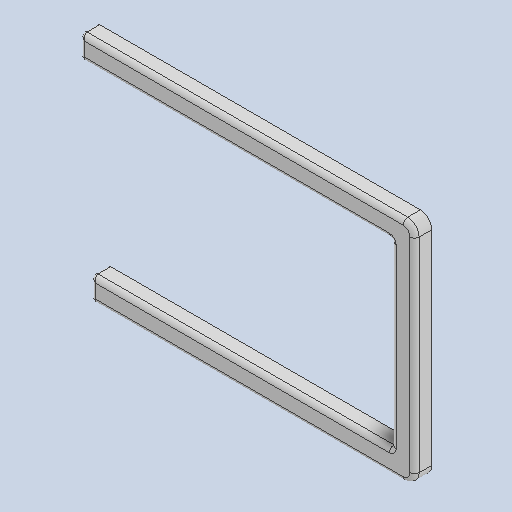
# Autodesk Inventor part: Top_Right
Saved by Autodesk Inventor 2023 (Build 270158000, 158)
## iProperties
Created: 2022-11-13
Part Number: Top_Right
Material: Generic
Document SubType Name: Modeling
Designer: reide
Density: 1 g/cm^3
Appearance: Default
Author: reide
Autodesk Inventor part; units mm, degrees
ref_plane "YZ Plane" through (0, 0, 0) normal (1, 0, 0) x (0, 1, 0)
ref_plane "XZ Plane" through (0, 0, 0) normal (0, 1, 0) x (-1, 0, 0)
ref_plane "XY Plane" through (0, 0, 0) normal (0, 0, 1) x (1, 0, 0)
sketch "Sketch1" plane through (0, 0, 0) normal (0, 0, 1) x (1, 0, 0)
  line L0 (-55.675, 43.6202) -> (-45.6, 43.6202)
  arc A0 (-46.5875, 44.4623) -> (-45.6, 43.6202) centre (-45.6, 44.6202) ccw
  ellipse E0 centre (-45.6, 44.2959) end of major axis (-45.6, 43.2418) minor radius 1 (-45.6, 45.35) -> (-46.5875, 44.4623) ccw
  line L1 (-45.6, 45.35) -> (-32.6, 45.35)
  ellipse E1 centre (-32.6, 44.2959) end of major axis (-32.6, 43.2418) minor radius 1 (-31.6, 44.2959) -> (-32.6, 45.35) ccw
  line L2 (-31.6, 42.35) -> (-31.6, 44.2959)
  arc A1 (-32.6, 41.35) -> (-31.6, 42.35) centre (-32.6, 42.35) ccw
  line L3 (-32.6, 41.35) -> (-37.675, 41.35)
  arc A2 (-38.675, 42.35) -> (-37.675, 41.35) centre (-37.675, 42.35) ccw
  line L4 (-38.675, 42.35) -> (-38.675, 40.35)
  arc A3 (-38.675, 40.35) -> (-37.675, 39.35) centre (-37.675, 40.35) ccw
  line L5 (-37.675, 39.35) -> (-31.6, 39.35)
  line L6 (-31.6, 39.35) -> (-31.6, 41.65)
  arc A4 (-30.6, 42.65) -> (-31.6, 41.65) centre (-30.6, 41.65) ccw
  line L7 (-30.6, 42.65) -> (-12, 42.65)
  arc A5 (-11, 41.65) -> (-12, 42.65) centre (-12, 41.65) ccw
  line L8 (-11, 41.65) -> (-11, 39.35)
  line L9 (-11, 39.35) -> (25.55, 39.35)
  line L10 (25.55, 39.35) -> (25.55, 41.65)
  arc A6 (26.55, 42.65) -> (25.55, 41.65) centre (26.55, 41.65) ccw
  line L11 (26.55, 42.65) -> (45.15, 42.65)
  arc A7 (46.15, 41.65) -> (45.15, 42.65) centre (45.15, 41.65) ccw
  line L12 (46.15, 41.65) -> (46.15, 39.35)
  line L13 (46.15, 39.35) -> (61.675, 39.35)
  arc A8 (62.675, 38.35) -> (61.675, 39.35) centre (61.675, 38.35) ccw
  line L14 (62.675, 38.35) -> (62.675, 15.986)
  arc A9 (62.675, 15.986) -> (63.675, 14.986) centre (63.675, 15.986) ccw
  line L15 (63.675, 14.986) -> (66.925, 14.986)
  line L16 (66.925, 14.986) -> (66.925, 14.8578)
  spline S0 degree 3 poles (66.925, 14.8578) (66.925, 14.7146) (66.9302, 14.5854) (66.9421, 14.2499) (66.9452, 14.1381) (66.9452, 13.986) knots 0 0 0 0 0.477344 0.477344 1 1 1 1
  line L17 (66.9452, 13.986) -> (66.9452, 2.986)
  spline S1 degree 3 poles (66.9452, 2.986) (66.9452, 2.8339) (66.9421, 2.7221) (66.9302, 2.3866) (66.925, 2.2574) (66.925, 2.1142) knots 0 0 0 0 0.522656 0.522656 1 1 1 1
  line L18 (66.925, 2.1142) -> (66.925, 1.986)
  line L19 (66.925, 1.986) -> (63.675, 1.986)
  arc A10 (63.675, 1.986) -> (62.675, 0.986) centre (63.675, 0.986) ccw
  line L20 (62.675, 0.986) -> (62.675, -2.225)
  line L21 (62.675, -2.225) -> (64.975, -2.225)
  arc A11 (65.975, -3.225) -> (64.975, -2.225) centre (64.975, -3.225) ccw
  line L22 (65.975, -3.225) -> (65.975, -21.825)
  arc A12 (64.975, -22.825) -> (65.975, -21.825) centre (64.975, -21.825) ccw
  line L23 (64.975, -22.825) -> (62.675, -22.825)
  line L24 (62.675, -22.825) -> (62.675, -38.35)
  arc A13 (61.675, -39.35) -> (62.675, -38.35) centre (61.675, -38.35) ccw
  line L25 (61.675, -39.35) -> (46.15, -39.35)
  line L26 (46.15, -39.35) -> (46.15, -41.65)
  arc A14 (45.15, -42.65) -> (46.15, -41.65) centre (45.15, -41.65) ccw
  line L27 (45.15, -42.65) -> (26.55, -42.65)
  arc A15 (25.55, -41.65) -> (26.55, -42.65) centre (26.55, -41.65) ccw
  line L28 (25.55, -41.65) -> (25.55, -39.35)
  line L29 (25.55, -39.35) -> (-31.2875, -39.35)
  line L30 (-31.2875, -39.35) -> (-31.2875, -41.65)
  arc A16 (-32.2875, -42.65) -> (-31.2875, -41.65) centre (-32.2875, -41.65) ccw
  line L31 (-32.2875, -42.65) -> (-50.8875, -42.65)
  arc A17 (-51.8875, -41.65) -> (-50.8875, -42.65) centre (-50.8875, -41.65) ccw
  line L32 (-51.8875, -41.65) -> (-51.8875, -39.35)
  line L33 (-51.8875, -39.35) -> (-66.9125, -39.35)
  arc A18 (-66.9125, -39.35) -> (-67.9125, -40.35) centre (-66.9125, -40.35) ccw
  line L34 (-67.9125, -40.35) -> (-67.9125, -48.35)
  arc A19 (-67.9125, -48.35) -> (-66.9125, -49.35) centre (-66.9125, -48.35) ccw
  line L35 (-66.9125, -49.35) -> (67.675, -49.35)
  arc A20 (67.675, -49.35) -> (72.675, -44.35) centre (67.675, -44.35) ccw
  line L36 (72.675, -44.35) -> (72.675, 44.35)
  arc A21 (72.675, 44.35) -> (67.675, 49.35) centre (67.675, 44.35) ccw
  line L37 (67.675, 49.35) -> (-71.675, 49.35)
  arc A22 (-71.675, 49.35) -> (-72.675, 48.35) centre (-71.675, 48.35) ccw
  line L38 (-72.675, 48.35) -> (-72.675, 40.35)
  arc A23 (-72.675, 40.35) -> (-71.675, 39.35) centre (-71.675, 40.35) ccw
  line L39 (-71.675, 39.35) -> (-57.675, 39.35)
  arc A24 (-57.675, 39.35) -> (-56.675, 40.35) centre (-57.675, 40.35) ccw
  line L40 (-56.675, 40.35) -> (-56.675, 43.6)
  line L41 (-56.675, 43.6) -> (-56.5468, 43.6)
  spline S2 degree 3 poles (-56.5468, 43.6) (-56.4036, 43.6) (-56.2744, 43.6052) (-55.9389, 43.6171) (-55.8271, 43.6202) (-55.675, 43.6202) knots 0 0 0 0 0.477344 0.477344 1 1 1 1
  line L42 (47.15, -41.35) -> (60.15, -41.35)
  arc A25 (61.15, -42.35) -> (60.15, -41.35) centre (60.15, -42.35) ccw
  line L43 (61.15, -44.2959) -> (61.15, -42.35)
  ellipse E2 centre (60.15, -44.2959) end of major axis (60.15, -43.2418) minor radius 1 (60.15, -45.35) -> (61.15, -44.2959) ccw
  line L44 (60.15, -45.35) -> (47.15, -45.35)
  ellipse E3 centre (47.15, -44.2959) end of major axis (47.15, -43.2418) minor radius 1 (46.15, -44.2959) -> (47.15, -45.35) ccw
  line L45 (46.15, -42.35) -> (46.15, -44.2959)
  arc A26 (47.15, -41.35) -> (46.15, -42.35) centre (47.15, -42.35) ccw
  line L46 (-30.2875, -41.35) -> (-17.2875, -41.35)
  arc A27 (-16.2875, -42.35) -> (-17.2875, -41.35) centre (-17.2875, -42.35) ccw
  line L47 (-16.2875, -44.2959) -> (-16.2875, -42.35)
  ellipse E4 centre (-17.2875, -44.2959) end of major axis (-17.2875, -43.2418) minor radius 1 (-17.2875, -45.35) -> (-16.2875, -44.2959) ccw
  line L48 (-17.2875, -45.35) -> (-30.2875, -45.35)
  ellipse E5 centre (-30.2875, -44.2959) end of major axis (-30.2875, -43.2418) minor radius 1 (-31.2875, -44.2959) -> (-30.2875, -45.35) ccw
  line L49 (-31.2875, -42.35) -> (-31.2875, -44.2959)
  arc A28 (-30.2875, -41.35) -> (-31.2875, -42.35) centre (-30.2875, -42.35) ccw
  circle A29 centre (-62.9125, -44.35) radius 2.125
  circle A30 centre (67.675, -44.35) radius 2.125
  circle A31 centre (-67.675, 44.35) radius 2.125
  circle A32 centre (67.675, 44.35) radius 2.125
  arc A33 (46.15, 42.35) -> (47.15, 41.35) centre (47.15, 42.35) ccw
  line L50 (46.15, 44.2959) -> (46.15, 42.35)
  ellipse E6 centre (47.15, 44.2959) end of major axis (47.15, 43.2418) minor radius 1 (47.15, 45.35) -> (46.15, 44.2959) ccw
  line L51 (47.15, 45.35) -> (60.15, 45.35)
  ellipse E7 centre (60.15, 44.2959) end of major axis (60.15, 43.2418) minor radius 1 (61.15, 44.2959) -> (60.15, 45.35) ccw
  line L52 (61.15, 42.35) -> (61.15, 44.2959)
  arc A34 (60.15, 41.35) -> (61.15, 42.35) centre (60.15, 42.35) ccw
  line L53 (60.15, 41.35) -> (47.15, 41.35)
  line L54 (-57.675, 39.35) -> (46.15, 39.35)
  line L55 (62.675, 15.986) -> (62.675, -22.825)
  line L56 (46.15, -39.35) -> (-51.8875, -39.35)
  point P0 (0, 0)
  constraints: 6 end point, 2 perpendicular, 1 horizontal, 8 other
extrude "Extrusion1" add sketch "Sketch1" along normal blind 7.5 contours S2 L41 L40 A24 L39 A23 L38 A22 L37 A21 L36 A20 L35 A19 L34 A18 L33 L32 A17 L31 A16 L30 L29 L28 A15 L27 A14 L26 L25 A13 L24 L23 A12 L22 A11 L21 L20 A10 L19 L18 S1 L17 S0 L16 L15 A9 L14 A8 L13 L12 A7 L11 A6 L10 L9 L8 A5 L7 A4 L6 L5 A3 L4 A2 L3 A1 L2 E1 L1 E0 A0 L0 | L0 A0 E0 L1 E1 L2 A1 L3 A2 L4 A3 L54 A24 L40 L41 S2 | L6 A4 L7 A5 L8 L54 | L10 A6 L11 A7 L12 L54 | A9 L15 L16 S0 L17 S1 L18 L19 A10 L55 | L21 A11 L22 A12 L23 L55 | L56 L30 A16 L31 A17 L32 | L26 A14 L27 A15 L28 L56 | L42 A25 L43 E2 L44 E3 L45 A26 | L46 A27 L47 E4 L48 E5 L49 A28 | A29 | A30 | A31 | A32 | L50 E6 L51 E7 L52 A34 L53 A33
fillet "Fillet1" radius 2 30 edges at (62.3821, 39.0571, 7.5) (62.675, -30.5875, 7.5) (62.675, -12.525, 7.5) (62.675, -0.6195, 7.5) (62.675, 8.486, 7.5) (62.675, 27.168, 7.5) (62.3821, -39.0571, 7.5) (-59.4, -39.35, 7.5) (-41.5875, -39.35, 7.5) (-2.8687, -39.35, 7.5) (35.85, -39.35, 7.5) (53.9125, -39.35, 7.5) (-67.6196, -39.6429, 7.5) (-67.9125, -44.35, 7.5) (-67.6196, -49.0571, 7.5) (0.3813, -49.35, 7.5) (71.2105, -47.8855, 7.5) (72.675, 0, 7.5) (71.2105, 47.8855, 7.5) (-2, 49.35, 7.5) (-72.3821, 49.0571, 7.5) (-72.675, 44.35, 7.5) (-72.3821, 39.6429, 7.5) (7.275, 39.35, 7.5) (-21.3, 39.35, 7.5) (-34.6375, 39.35, 7.5) (-47.675, 39.35, 7.5) (-64.675, 39.35, 7.5) (53.9125, 39.35, 7.5) (35.85, 39.35, 7.5)
sketch "Sketch3" plane through (-72.675, 40.35, 0) normal (-1, 0, 0) x (0, 0, 1)
  line L0 (0, -40.35) -> (17.2642, -40.35)
  line L1 (0.1, -1) -> (5.6, -1) projected
  line L2 (0.1, 9) -> (5.6, 9) projected
  line L3 (0, -84.7) -> (0, 4) projected
  line L4 (0, -1) -> (5.5, -1) projected
  line L5 (0, -1) -> (0, 1)
  line L6 (0, 1) -> (3, 1)
  line L7 (3, 1) -> (3, 6.3)
  line L8 (0, 1) -> (0, 5.3)
  line L9 (0, 5.3) -> (3, 6.3)
  line L10 (0.1, -79.7) -> (5.6, -79.7)
  line L11 (0, 4) -> (0, -84.7)
  line L12 (0, -79.7) -> (5.5, -79.7)
  line L13 (0, -79.7) -> (0, -81.7)
  line L14 (0, -81.7) -> (3, -81.7)
  line L15 (3, -81.7) -> (3, -87)
  line L16 (0, -81.7) -> (0, -86)
  line L17 (0, -82.575) -> (0, -86.825)
  line L18 (0, -86) -> (3, -87)
  point P0 (0, 1.875)
  point P1 (0, 1)
  dimension "d11" = 2
  dimension "d12" = 3
  dimension "d13" = 5.3
  dimension "d14" = 4.3
  constraints: 30 end point, 11 symmetric about line, 1 horizontal, 1 perpendicular, 1 point on line, 1 vertical
  measures "d11" distance of L4.start L5.end
  measures "d12" distance of L5.end L6.end
  measures "d13" distance of L6.end L7.end
  measures "d14" distance of L5.end L8.end
extrude "Extrusion3" cut sketch "Sketch3" against normal up to surface (145.35 mm away)
sketch "Sketch4" plane through (0, 0, 0) normal (0, 0, -1) x (-1, 0, 0)
  line L0 (55.675, 43.605) -> (45.6, 43.605)
  arc A0 (45.6, 43.605) -> (46.5886, 44.4545) centre (45.6, 44.605) ccw
  ellipse E0 centre (45.6, 44.2959) end of major axis (45.6, 43.2418) minor radius 1 (46.5886, 44.4545) -> (45.6, 45.35) ccw
  line L1 (45.6, 45.35) -> (32.6, 45.35)
  ellipse E1 centre (32.6, 44.2959) end of major axis (32.6, 43.2418) minor radius 1 (32.6, 45.35) -> (31.6, 44.2959) ccw
  line L2 (31.6, 42.35) -> (31.6, 44.2959)
  arc A1 (31.6, 42.35) -> (32.6, 41.35) centre (32.6, 42.35) ccw
  line L3 (32.6, 41.35) -> (37.675, 41.35)
  arc A2 (37.675, 41.35) -> (38.675, 42.35) centre (37.675, 42.35) ccw
  line L4 (38.675, 42.35) -> (38.675, 40.35)
  arc A3 (37.675, 39.35) -> (38.675, 40.35) centre (37.675, 40.35) ccw
  line L5 (37.675, 39.35) -> (31.6, 39.35)
  line L6 (31.6, 39.35) -> (31.6, 41.65)
  arc A4 (31.6, 41.65) -> (30.6, 42.65) centre (30.6, 41.65) ccw
  line L7 (30.6, 42.65) -> (12, 42.65)
  arc A5 (12, 42.65) -> (11, 41.65) centre (12, 41.65) ccw
  line L8 (11, 41.65) -> (11, 39.35)
  line L9 (11, 39.35) -> (-25.55, 39.35)
  line L10 (-25.55, 39.35) -> (-25.55, 41.65)
  arc A6 (-25.55, 41.65) -> (-26.55, 42.65) centre (-26.55, 41.65) ccw
  line L11 (-26.55, 42.65) -> (-45.15, 42.65)
  arc A7 (-45.15, 42.65) -> (-46.15, 41.65) centre (-45.15, 41.65) ccw
  line L12 (-46.15, 41.65) -> (-46.15, 39.35)
  line L13 (-46.15, 39.35) -> (-61.675, 39.35)
  arc A8 (-61.675, 39.35) -> (-62.675, 38.35) centre (-61.675, 38.35) ccw
  line L14 (-62.675, 38.35) -> (-62.675, 15.986)
  arc A9 (-63.675, 14.986) -> (-62.675, 15.986) centre (-63.675, 15.986) ccw
  line L15 (-63.675, 14.986) -> (-66.925, 14.986)
  line L16 (-66.925, 14.986) -> (-66.925, 14.6105)
  spline S0 degree 3 poles (-66.925, 14.6105) (-66.925, 14.5088) (-66.9263, 14.4189) (-66.9292, 14.1781) (-66.93, 14.0946) (-66.93, 13.986) knots 0 0 0 0 0.491042 0.491042 1 1 1 1
  line L17 (-66.93, 13.986) -> (-66.93, 2.986)
  spline S1 degree 3 poles (-66.93, 2.986) (-66.93, 2.8774) (-66.9292, 2.7939) (-66.9263, 2.5531) (-66.925, 2.4632) (-66.925, 2.3615) knots 0 0 0 0 0.508958 0.508958 1 1 1 1
  line L18 (-66.925, 2.3615) -> (-66.925, 1.986)
  line L19 (-66.925, 1.986) -> (-63.675, 1.986)
  arc A10 (-62.675, 0.986) -> (-63.675, 1.986) centre (-63.675, 0.986) ccw
  line L20 (-62.675, 0.986) -> (-62.675, -2.225)
  line L21 (-62.675, -2.225) -> (-64.975, -2.225)
  arc A11 (-64.975, -2.225) -> (-65.975, -3.225) centre (-64.975, -3.225) ccw
  line L22 (-65.975, -3.225) -> (-65.975, -21.825)
  arc A12 (-65.975, -21.825) -> (-64.975, -22.825) centre (-64.975, -21.825) ccw
  line L23 (-64.975, -22.825) -> (-62.675, -22.825)
  line L24 (-62.675, -22.825) -> (-62.675, -38.35)
  arc A13 (-62.675, -38.35) -> (-61.675, -39.35) centre (-61.675, -38.35) ccw
  line L25 (-61.675, -39.35) -> (-46.15, -39.35)
  line L26 (-46.15, -39.35) -> (-46.15, -41.65)
  arc A14 (-46.15, -41.65) -> (-45.15, -42.65) centre (-45.15, -41.65) ccw
  line L27 (-45.15, -42.65) -> (-26.55, -42.65)
  arc A15 (-26.55, -42.65) -> (-25.55, -41.65) centre (-26.55, -41.65) ccw
  line L28 (-25.55, -41.65) -> (-25.55, -39.35)
  line L29 (-25.55, -39.35) -> (31.2875, -39.35)
  line L30 (31.2875, -39.35) -> (31.2875, -41.65)
  arc A16 (31.2875, -41.65) -> (32.2875, -42.65) centre (32.2875, -41.65) ccw
  line L31 (32.2875, -42.65) -> (50.8875, -42.65)
  arc A17 (50.8875, -42.65) -> (51.8875, -41.65) centre (50.8875, -41.65) ccw
  line L32 (51.8875, -41.65) -> (51.8875, -39.35)
  line L33 (51.8875, -39.35) -> (66.9125, -39.35)
  arc A18 (67.9125, -40.35) -> (66.9125, -39.35) centre (66.9125, -40.35) ccw
  line L34 (67.9125, -40.35) -> (67.9125, -48.35)
  arc A19 (66.9125, -49.35) -> (67.9125, -48.35) centre (66.9125, -48.35) ccw
  line L35 (66.9125, -49.35) -> (-67.675, -49.35)
  arc A20 (-72.675, -44.35) -> (-67.675, -49.35) centre (-67.675, -44.35) ccw
  line L36 (-72.675, -44.35) -> (-72.675, 44.35)
  arc A21 (-67.675, 49.35) -> (-72.675, 44.35) centre (-67.675, 44.35) ccw
  line L37 (-67.675, 49.35) -> (71.675, 49.35)
  arc A22 (72.675, 48.35) -> (71.675, 49.35) centre (71.675, 48.35) ccw
  line L38 (72.675, 48.35) -> (72.675, 40.35)
  arc A23 (71.675, 39.35) -> (72.675, 40.35) centre (71.675, 40.35) ccw
  line L39 (71.675, 39.35) -> (57.675, 39.35)
  arc A24 (56.675, 40.35) -> (57.675, 39.35) centre (57.675, 40.35) ccw
  line L40 (56.675, 40.35) -> (56.675, 43.6)
  line L41 (56.675, 43.6) -> (56.2995, 43.6)
  spline S2 degree 3 poles (56.2995, 43.6) (56.1978, 43.6) (56.1079, 43.6013) (55.8671, 43.6042) (55.7836, 43.605) (55.675, 43.605) knots 0 0 0 0 0.491042 0.491042 1 1 1 1
  line L42 (-47.15, -41.3502) -> (-60.15, -41.3502)
  arc A25 (-60.15, -41.3502) -> (-61.15, -42.3502) centre (-60.15, -42.3502) ccw
  line L43 (-61.15, -44.2961) -> (-61.15, -42.3502)
  ellipse E2 centre (-60.15, -44.2961) end of major axis (-60.15, -43.242) minor radius 1 (-61.15, -44.2961) -> (-60.15, -45.3502) ccw
  line L44 (-60.15, -45.3502) -> (-47.15, -45.3502)
  ellipse E3 centre (-47.15, -44.2961) end of major axis (-47.15, -43.242) minor radius 1 (-47.15, -45.3502) -> (-46.15, -44.2961) ccw
  line L45 (-46.15, -42.3502) -> (-46.15, -44.2961)
  arc A26 (-46.15, -42.3502) -> (-47.15, -41.3502) centre (-47.15, -42.3502) ccw
  line L46 (30.2875, -41.3502) -> (17.2875, -41.3502)
  arc A27 (17.2875, -41.3502) -> (16.2875, -42.3502) centre (17.2875, -42.3502) ccw
  line L47 (16.2875, -44.2961) -> (16.2875, -42.3502)
  ellipse E4 centre (17.2875, -44.2961) end of major axis (17.2875, -43.242) minor radius 1 (16.2875, -44.2961) -> (17.2875, -45.3502) ccw
  line L48 (17.2875, -45.3502) -> (30.2875, -45.3502)
  ellipse E5 centre (30.2875, -44.2961) end of major axis (30.2875, -43.242) minor radius 1 (30.2875, -45.3502) -> (31.2875, -44.2961) ccw
  line L49 (31.2875, -42.3502) -> (31.2875, -44.2961)
  arc A28 (31.2875, -42.3502) -> (30.2875, -41.3502) centre (30.2875, -42.3502) ccw
  circle A29 centre (62.9125, -44.35) radius 2.125
  circle A30 centre (-67.675, -44.35) radius 2.125
  circle A31 centre (67.675, 44.35) radius 2.125
  circle A32 centre (-67.675, 44.35) radius 2.125
  arc A33 (-47.15, 41.35) -> (-46.15, 42.35) centre (-47.15, 42.35) ccw
  line L50 (-46.15, 44.2959) -> (-46.15, 42.35)
  ellipse E6 centre (-47.15, 44.2959) end of major axis (-47.15, 43.2418) minor radius 1 (-46.15, 44.2959) -> (-47.15, 45.35) ccw
  line L51 (-47.15, 45.35) -> (-60.15, 45.35)
  ellipse E7 centre (-60.15, 44.2959) end of major axis (-60.15, 43.2418) minor radius 1 (-60.15, 45.35) -> (-61.15, 44.2959) ccw
  line L52 (-61.15, 42.35) -> (-61.15, 44.2959)
  arc A34 (-61.15, 42.35) -> (-60.15, 41.35) centre (-60.15, 42.35) ccw
  line L53 (-60.15, 41.35) -> (-47.15, 41.35)
  arc A35 (-72.675, -44.35) -> (-72.1146, -46.65) centre (-67.675, -44.35) ccw
  line L54 (67.9125, -46.65) -> (-72.1146, -46.65)
  line L55 (67.9125, -41.35) -> (67.9125, -46.65)
  line L56 (67.9125, -41.35) -> (-72.675, -41.35)
  line L57 (-72.675, -44.35) -> (-72.675, -41.35)
  arc A36 (-72.1146, 46.65) -> (-72.675, 44.35) centre (-67.675, 44.35) ccw
  line L58 (-72.675, 41.35) -> (-72.675, 44.35)
  line L59 (72.675, 41.35) -> (-72.675, 41.35)
  line L60 (72.675, 46.65) -> (72.675, 41.35)
  line L61 (72.675, 46.65) -> (-72.1146, 46.65)
  line L62 (16.2875, -46.65) -> (47.2875, -46.65)
  line L63 (47.2875, -46.65) -> (47.2875, -41.35)
  line L64 (47.2875, -41.35) -> (16.2875, -41.35)
  line L65 (16.2875, -41.35) -> (16.2875, -46.65)
  line L66 (-61.15, -41.35) -> (-30.15, -41.35)
  line L67 (-30.15, -41.35) -> (-30.15, -46.65)
  line L68 (-30.15, -46.65) -> (-61.15, -46.65)
  line L69 (-61.15, -46.65) -> (-61.15, -41.35)
  line L70 (31.5804, 46.65) -> (62.5804, 46.65)
  line L71 (62.5804, 46.65) -> (62.5804, 41.35)
  line L72 (62.5804, 41.35) -> (31.5804, 41.35)
  line L73 (31.5804, 41.35) -> (31.5804, 46.65)
  line L74 (-61.15, 46.65) -> (-30.15, 46.65)
  line L75 (-30.15, 46.65) -> (-30.15, 41.35)
  line L76 (-30.15, 41.35) -> (-61.15, 41.35)
  line L77 (-61.15, 41.35) -> (-61.15, 46.65)
  point P0 (0, 0)
  point P1 (-30.15, 44)
  point P2 (-61.15, 43.323)
  point P3 (-61.15, 44)
  point P4 (16.2875, -42.3502)
  dimension "d15" = 31
  dimension "d16" = 31
  dimension "d17" = 31
  dimension "d18" = 31
  dimension "d19" = 0
  constraints: 32 end point, 9 point on line, 8 parallel, 4 horizontal, 4 perpendicular, 3 midpoint, 8 other
  measures "d15" distance between parallel lines of L65 L63
  measures "d16" distance between parallel lines of L69 L67
  measures "d17" distance between parallel lines of L73 L71
  measures "d18" distance from line of L77 point (-30.15, 44)
  measures "d19" horizontal distance of point (-61.15, 43.323) point (-61.15, 44)
extrude "Extrusion4" add sketch "Sketch4" against normal up to surface (3 mm away) contours L71 L61 L38 L59 | L73 A4 L7 A5 L8 L59 L10 A6 L11 L75 L61 | L73 L59 L8 A5 L7 A4 | L77 L52 L59 L36 A21 L61 | L11 A6 L10 L59 L75 | L56 L69 L43 L54 A20 L36 | L67 L27 A15 L28 L56 L65 L47 L54 | L67 L56 L28 A15 L27 | L54 L63 L31 A17 L32 L56 L34 | L63 L56 L32 A17 L31 | A29 | A30 | A31 | A32
sketch "Sketch5" plane through (0, 0, 0) normal (0, 0, -1) x (-1, 0, 0)
  line L0 (47.2875, -46.65) -> (47.2875, -41.35) projected
  line L1 (47.2875, -41.35) -> (16.2875, -41.35) projected
  line L2 (16.2875, -41.35) -> (16.2875, -46.65) projected
  line L3 (47.2875, -46.65) -> (16.2875, -46.65) projected
  line L4 (-61.15, -41.35) -> (-61.15, -46.65) projected
  line L5 (-30.15, -46.65) -> (-61.15, -46.65) projected
  line L6 (-30.15, -46.65) -> (-30.15, -41.35) projected
  line L7 (-30.15, -41.35) -> (-61.15, -41.35) projected
  line L8 (-30.15, 41.35) -> (-30.15, 46.65) projected
  line L9 (-30.15, 46.65) -> (-61.15, 46.65) projected
  line L10 (-61.15, 46.65) -> (-61.15, 41.35) projected
  line L11 (-30.15, 41.35) -> (-61.15, 41.35) projected
  line L12 (31.5804, 46.65) -> (31.5804, 41.35) projected
  line L13 (62.5804, 41.35) -> (31.5804, 41.35) projected
  line L14 (62.5804, 41.35) -> (62.5804, 46.65) projected
  line L15 (62.5804, 46.65) -> (31.5804, 46.65) projected
  arc A0 (-67.675, -49.35) -> (-72.675, -44.35) centre (-67.675, -44.35) ccw projected
  line L16 (66.9125, -49.35) -> (-67.675, -49.35) projected
  arc A1 (66.9125, -49.35) -> (67.9125, -48.35) centre (66.9125, -48.35) ccw projected
  line L17 (67.9125, -40.35) -> (67.9125, -48.35) projected
  arc A2 (67.9125, -40.35) -> (66.9125, -39.35) centre (66.9125, -40.35) ccw projected
  line L18 (-61.675, -39.35) -> (66.9125, -39.35) projected
  arc A3 (-62.675, -38.35) -> (-61.675, -39.35) centre (-61.675, -38.35) ccw projected
  line L19 (-62.675, 38.35) -> (-62.675, -38.35) projected
  arc A4 (-61.675, 39.35) -> (-62.675, 38.35) centre (-61.675, 38.35) ccw projected
  line L20 (71.675, 39.35) -> (-61.675, 39.35) projected
  arc A5 (71.675, 39.35) -> (72.675, 40.35) centre (71.675, 40.35) ccw projected
  line L21 (72.675, 48.35) -> (72.675, 40.35) projected
  arc A6 (72.675, 48.35) -> (71.675, 49.35) centre (71.675, 48.35) ccw projected
  line L22 (-67.675, 49.35) -> (71.675, 49.35) projected
  arc A7 (-67.675, 49.35) -> (-72.675, 44.35) centre (-67.675, 44.35) ccw projected
  line L23 (-72.675, -44.35) -> (-72.675, 44.35) projected
  line L24 (-61.15, -45.65) -> (-61.15, -41.35) projected
  line L25 (-61.15, -41.35) -> (-30.15, -41.35) projected
  line L26 (-30.15, -41.35) -> (-30.15, -45.65) projected
  line L27 (-30.15, -45.65) -> (-61.15, -45.65) projected
  line L28 (31.5804, 45.65) -> (62.5804, 45.65) projected
  line L29 (62.5804, 45.65) -> (62.5804, 41.35) projected
  line L30 (62.5804, 41.35) -> (31.5804, 41.35) projected
  line L31 (31.5804, 41.35) -> (31.5804, 45.65) projected
  line L32 (-30.15, 45.65) -> (-30.15, 41.35) projected
  line L33 (-30.15, 41.35) -> (-61.15, 41.35) projected
  line L34 (-61.15, 41.35) -> (-61.15, 45.65) projected
  line L35 (-61.15, 45.65) -> (-30.15, 45.65) projected
  line L36 (47.2875, -41.35) -> (47.2875, -45.65) projected
  line L37 (47.2875, -45.65) -> (16.2875, -45.65) projected
  line L38 (16.2875, -45.65) -> (16.2875, -41.35) projected
  line L39 (16.2875, -41.35) -> (47.2875, -41.35) projected
  line L40 (16.2875, -41.35) -> (31.2875, -41.35)
  line L41 (31.2875, -41.35) -> (31.2875, -46.65)
  line L42 (31.2875, -46.65) -> (16.2875, -46.65)
  line L43 (16.2875, -46.65) -> (16.2875, -41.35)
  line L44 (-61.15, -46.65) -> (-46.15, -46.65)
  line L45 (-46.15, -46.65) -> (-46.15, -41.35)
  line L46 (-46.15, -41.35) -> (-61.15, -41.35)
  line L47 (-61.15, -41.35) -> (-61.15, -46.65)
  line L48 (-61.15, 46.65) -> (-46.15, 46.65)
  line L49 (-46.15, 46.65) -> (-46.15, 41.35)
  line L50 (-46.15, 41.35) -> (-61.15, 41.35)
  line L51 (-61.15, 41.35) -> (-61.15, 46.65)
  line L52 (31.5804, 46.65) -> (46.5804, 46.65)
  line L53 (46.5804, 46.65) -> (46.5804, 41.35)
  line L54 (46.5804, 41.35) -> (31.5804, 41.35)
  line L55 (31.5804, 41.35) -> (31.5804, 46.65)
  point P0 (0, 0)
  point P1 (16.2875, -43.5)
  dimension "d22" = 15
  dimension "d23" = 15
  dimension "d24" = 15
  dimension "d25" = 15
  constraints: 32 end point, 8 parallel, 4 horizontal, 4 perpendicular, 4 point on line, 1 midpoint
  measures "d22" distance from line of point (16.287, -43.5) L41
  measures "d23" distance of L46.end L45.end
  measures "d24" distance of L49.end L50.end
  measures "d25" distance of L53.end L54.end
extrude "Extrusion5" cut sketch "Sketch5" against normal up to surface (3 mm away) contours L3 L41 L37 L0 | L37 L41 L1 L0 | L7 L6 L27 L45 | L27 L6 L5 L45 | L11 L49 L35 L8 | L35 L49 L9 L8 | L15 L14 L28 L53 | L28 L14 L13 L53
sketch "Sketch6" plane through (0, 0, 0) normal (0, 0, -1) x (-1, 0, 0)
  circle A0 centre (67.675, 44.35) radius 2.125 projected
  circle A1 centre (-67.675, 44.35) radius 2.125 projected
  circle A2 centre (-67.675, -44.35) radius 2.125 projected
  circle A3 centre (62.9125, -44.35) radius 2.125 projected
  point P0 (0, 0)
extrude "Extrusion6" cut sketch "Sketch6" against normal blind 1.8
body "Solid1"
